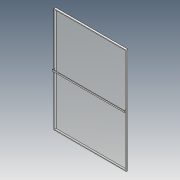
# Autodesk Inventor part: SlidingDoorPanel
Saved by Autodesk Inventor 2018.3 (Build 223284000, 284)
## iProperties
Created: 2019-11-06
Part Number: SlidingDoorPanel
Material: Generic
Document SubType Name: Modeling
Designer: MattBussey
Density: 1 g/cm^3
Appearance: Default
RuleStatus: InUse
Author: MattBussey
Autodesk Inventor part; units mm, degrees
ref_plane "YZ Plane" through (0, 0, 0) normal (1, 0, 0) x (0, 1, 0)
sketch "Sketch1" plane through (0, 0, 0) normal (0, 0, 1) x (1, 0, 0)
  line L0 (0, 0) -> (1536.7, 0)
  line L1 (1536.7, 0) -> (1536.7, 2235.2)
  line L2 (1536.7, 2235.2) -> (0, 2235.2)
  line L3 (0, 2235.2) -> (0, 0)
  line L4 (12.7, 2222.5) -> (1524, 2222.5)
  line L5 (1524, 2222.5) -> (1524, 12.7)
  line L6 (1524, 12.7) -> (12.7, 12.7)
  line L7 (12.7, 12.7) -> (12.7, 2222.5)
  dimension "d2" = 2235.2
  dimension "d3" = 1536.7
  dimension "d4" = 12.7
  constraints: 16 end point, 4 parallel, 2 perpendicular, 1 horizontal, 3 other
  measures "d2" distance of L0.end L1.end
  measures "d3" distance of L0.start L0.end
  measures "d4" distance between parallel lines of L2 L4
extrude "GlassPane" add sketch "Sketch1" along normal blind 38.1 contours L4 L5 L6 L7
extrude "Frame" add sketch "Sketch1" along normal blind 38.1 separate body
ref_plane "Work Plane1" through (0, 1117.6, 0) normal (0, 1, 0) x (1, 0, 0)
ref_plane "Work Plane2" through (0, 0, 19.05) normal (0, 0, 1) x (1, 0, 0)
sketch "Sketch2" plane through (0, 1117.6, 0) normal (0, 1, 0) x (1, 0, 0)
  line L0 (12.7, -38.1) -> (0, -38.1)
  line L1 (0, -38.1) -> (0, -76.2)
  line L2 (0, -76.2) -> (1536.7, -76.2)
  line L3 (1536.7, -76.2) -> (1536.7, -38.1)
  line L4 (1536.7, -38.1) -> (1524, -38.1)
  line L5 (1524, -38.1) -> (1524, -63.5)
  line L6 (1524, -63.5) -> (12.7, -63.5)
  line L7 (12.7, -63.5) -> (12.7, -38.1)
  dimension "d7" = 12.7
  dimension "d8" = 12.7
  dimension "d9" = 38.1
  constraints: 16 end point, 5 perpendicular, 1 horizontal, 1 parallel
  measures "d7" distance between parallel lines of L7 L1
  measures "d8" distance between parallel lines of L6 L2
  measures "d9" distance from line of L0.end L2
extrude "Handle" add sketch "Sketch2" along normal mid plane 25.4 separate body
mirror "MirrorExterior" [suppressed]
equation "\"d2\" = Height - FrameWidth"
equation "\"d0\" = 0.375 * Depth"
equation "\"d5\" = 0.375 * Depth"
equation "\"d8\" = d7"
equation "\"Width\" = 3048"
equation "\"Height\" = 2286"
equation "\"Depth\" = 101.6"
equation "\"FrameWidth\" = 50.8"
